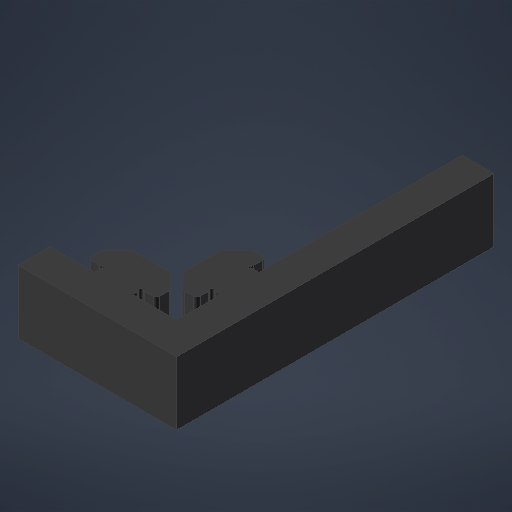
# Autodesk Inventor part: Guia_Perfil_test
Saved by Autodesk Inventor 2026.1 (Build 301233020, 233B)
## iProperties
Created: 2025-10-26
Part Number: Guia_Perfil_test
Material: Generic
Document SubType Name: Modeling
Designer: Tito Luyo Murata
Density: 1 g/cm^3
Appearance: Default
Author: Tito Luyo Murata
Autodesk Inventor part; units mm, degrees
ref_plane "YZ Plane" through (0, 0, 0) normal (1, 0, 0) x (0, 1, 0)
ref_plane "XZ Plane" through (0, 0, 0) normal (0, 1, 0) x (-1, 0, 0)
ref_plane "XY Plane" through (0, 0, 0) normal (0, 0, 1) x (1, 0, 0)
sketch "Sketch1" plane through (0, 0, 0) normal (0, 1, 0) x (-1, 0, 0)
  line L0 (0, 0) -> (5, 0)
  line L1 (5, -5) -> (5, -50)
  line L2 (5, -50) -> (0, -50)
  line L3 (0, -50) -> (0, 0)
  line L4 (0, 0) -> (25, 0)
  line L5 (25, 0) -> (25, -5)
  line L6 (25, -5) -> (5, -5)
  line L7 (12, -5) -> (18, -5)
  line L8 (18, -5) -> (18, -5.841)
  line L9 (17.75, -6.4) -> (12.25, -6.4)
  line L10 (12, -5.841) -> (12, -5)
  line L11 (20.4, -6.9) -> (20.4, -8.4363)
  line L12 (20.4, -8.65) -> (9.6, -8.65)
  line L13 (9.6, -8.4363) -> (9.6, -6.9)
  line L14 (17.95, -8.65) -> (12.05, -8.65)
  line L15 (12.05, -8.65) -> (12.05, -10.9932)
  line L16 (12.2506, -10.9932) -> (17.7494, -10.9932)
  line L17 (17.95, -10.9932) -> (17.95, -8.65)
  line L18 (9.7544, -8.7977) -> (11.905, -10.8545)
  line L19 (20.2456, -8.7977) -> (18.095, -10.8545)
  line L20 (0, 0) -> (21.2132, -21.2132) construction
  line L21 (0, 0) -> (30, 0) construction
  line L22 (18, -6.4) -> (12, -5) construction
  line L23 (18, -5) -> (12, -6.4) construction
  line L24 (20.4, -6.4) -> (9.6, -8.65) construction
  line L25 (20.4, -8.65) -> (9.6, -6.4) construction
  line L26 (15, -5.7) -> (15, -19.5518) construction
  line L27 (17.95, -8.65) -> (12.05, -10.9932) construction
  line L28 (12.05, -8.65) -> (17.95, -10.9932) construction
  arc A0 (10.1, -6.4) -> (9.6, -6.9) centre (10.1, -6.9) ccw
  arc A1 (9.6, -8.4363) -> (9.7544, -8.7977) centre (10.1, -8.4363) ccw
  arc A2 (11.905, -10.8545) -> (12.2506, -10.9932) centre (12.2506, -10.4932) ccw
  arc A3 (17.7494, -10.9932) -> (18.095, -10.8545) centre (17.7494, -10.4932) ccw
  arc A4 (20.2456, -8.7977) -> (20.4, -8.4363) centre (19.9, -8.4363) ccw
  arc A5 (20.4, -6.9) -> (19.9, -6.4) centre (19.9, -6.9) ccw
  arc A6 (11.8137, -6.5667) -> (12.1667, -6.2137) centre (12, -6.4) ccw
  arc A7 (17.8333, -6.2137) -> (18.1863, -6.5667) centre (18, -6.4) ccw
  line L29 (10.1, -6.4) -> (11.441, -6.4)
  line L30 (12.25, -6.4) -> (17.75, -6.4)
  line L31 (18.559, -6.4) -> (19.9, -6.4)
  arc A8 (12, -5.841) -> (12.1667, -6.2137) centre (12.5, -5.841) ccw
  arc A9 (11.8137, -6.5667) -> (11.441, -6.4) centre (11.441, -6.9) ccw
  arc A10 (17.8333, -6.2137) -> (18, -5.841) centre (17.5, -5.841) ccw
  arc A11 (18.559, -6.4) -> (18.1863, -6.5667) centre (18.559, -6.9) ccw
  line L32 (5, -12) -> (5, -18)
  line L33 (5, -18) -> (5.841, -18)
  line L34 (6.4, -17.75) -> (6.4, -12.25)
  line L35 (5.841, -12) -> (5, -12)
  line L36 (6.9, -20.4) -> (8.4363, -20.4)
  line L37 (8.65, -20.4) -> (8.65, -9.6)
  line L38 (8.4363, -9.6) -> (6.9, -9.6)
  line L39 (8.65, -17.95) -> (8.65, -12.05)
  line L40 (8.65, -12.05) -> (10.9932, -12.05)
  line L41 (10.9932, -12.2506) -> (10.9932, -17.7494)
  line L42 (10.9932, -17.95) -> (8.65, -17.95)
  line L43 (8.7977, -9.7544) -> (10.8545, -11.905)
  line L44 (8.7977, -20.2456) -> (10.8545, -18.095)
  line L45 (6.4, -18) -> (5, -12) construction
  line L46 (5, -18) -> (6.4, -12) construction
  line L47 (6.4, -20.4) -> (8.65, -9.6) construction
  line L48 (8.65, -20.4) -> (6.4, -9.6) construction
  line L49 (8.65, -17.95) -> (10.9932, -12.05) construction
  line L50 (8.65, -12.05) -> (10.9932, -17.95) construction
  arc A12 (6.9, -9.6) -> (6.4, -10.1) centre (6.9, -10.1) ccw
  arc A13 (8.7977, -9.7544) -> (8.4363, -9.6) centre (8.4363, -10.1) ccw
  arc A14 (10.9932, -12.2506) -> (10.8545, -11.905) centre (10.4932, -12.2506) ccw
  arc A15 (10.8545, -18.095) -> (10.9932, -17.7494) centre (10.4932, -17.7494) ccw
  arc A16 (8.4363, -20.4) -> (8.7977, -20.2456) centre (8.4363, -19.9) ccw
  arc A17 (6.4, -19.9) -> (6.9, -20.4) centre (6.9, -19.9) ccw
  arc A18 (6.2137, -12.1667) -> (6.5667, -11.8137) centre (6.4, -12) ccw
  arc A19 (6.5667, -18.1863) -> (6.2137, -17.8333) centre (6.4, -18) ccw
  line L51 (6.4, -10.1) -> (6.4, -11.441)
  line L52 (6.4, -12.25) -> (6.4, -17.75)
  line L53 (6.4, -18.559) -> (6.4, -19.9)
  arc A20 (6.2137, -12.1667) -> (5.841, -12) centre (5.841, -12.5) ccw
  arc A21 (6.4, -11.441) -> (6.5667, -11.8137) centre (6.9, -11.441) ccw
  arc A22 (5.841, -18) -> (6.2137, -17.8333) centre (5.841, -17.5) ccw
  arc A23 (6.5667, -18.1863) -> (6.4, -18.559) centre (6.9, -18.559) ccw
  point P0 (18, -5)
  point P1 (25.5, -11.3)
  point P2 (15, -7.525)
  point P3 (15, -9.8216)
  point P4 (9.648, -8.65)
  point P5 (20.352, -8.65)
  point P6 (11.75, -6.4)
  point P7 (12, -6.15)
  point P8 (18.25, -6.4)
  point P9 (18, -6.15)
  point P10 (5.7, -15)
  point P11 (7.525, -15)
  point P12 (9.8216, -15)
  point P13 (6.4, -11.75)
  point P14 (6.15, -12)
  point P15 (6.4, -18.25)
  point P16 (6.15, -18)
  dimension "d0" = 5
  dimension "d1" = 50
  dimension "d3" = 5
  dimension "d4" = 6
  dimension "d5" = 1.4
  dimension "d6" = 10.8
  dimension "d7" = 2.25
  dimension "d10" = 5.9
  dimension "d11" = 2.3432
  dimension "d13" = 25
  dimension "d14" = 30
  dimension "d15" = 45
  dimension "d18" = 7
  dimension "d20" = 0.5
  dimension "d21" = 0.5
  dimension "d22" = 0.5
  dimension "d23" = 0.5
  constraints: 108 end point, 60 point on circle, 53 symmetric about line, 35 point on line, 24 centre point, 24 tangent, 11 parallel, 8 equal radius, 8 horizontal, 7 perpendicular, 4 coincident, 3 midpoint, 1 equal length, 1 vertical, 12 other
  measures "d0" distance of L1.end L2.end
  measures "d1" distance of L0.end L1.end
  measures "d3" distance of L4.end L5.end
  measures "d4" distance of L22.start L23.end
  measures "d5" distance of L7.end L22.start
  measures "d6" distance of L12.start L12.end
  measures "d7" distance of L24.start L12.start
  measures "d10" distance of L17.start L15.end
  measures "d11" distance of L15.end L14.end
  measures "d13" distance of L0.start L4.end
  measures "d14" distance of L0.start L20.end
  measures "d15" angle of L20 L21
  measures "d18" distance between parallel lines of L1 L10
  measures "d20" radius of A0
  measures "d21" diameter of A6
  measures "d22" diameter of A7
  measures "d23" radius of A8
extrude "Extrusion1" add sketch "Sketch1" along normal blind 10
equation "\"d0\" = grosor"
equation "\"d3\" = grosor"
equation "\"d4\" = guia_cuello"
equation "\"d5\" = guia_sep_de_ext"
equation "\"d6\" = guia_ancho"
equation "\"d7\" = guia_ancho_espesor"
equation "\"d10\" = guia_ancho_menor"
equation "\"d11\" = guia_ancho_menor_espesor"
equation "\"d18\" = guia_sep_borde"
equation "\"grosor\" = 5"
equation "\"guia_tol\" = 0.1"
equation "\"guia_cuello\" = 6"
equation "\"guia_sep_de_ext\" = 1.4"
equation "\"guia_ancho\" = 10.8"
equation "\"guia_ancho_espesor\" = 2.25"
equation "\"guia_ancho_menor\" = 5.9"
equation "\"guia_ancho_menor_espesor\" = 2.343174"
equation "\"guia_sep_borde\" = 7"
body "Solid1"
